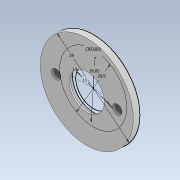
# Autodesk Inventor part: Sensor_AbstandFlansch
Saved by Autodesk Inventor 2022 (Build 260153000, 153)
## iProperties
Created: 2022-10-10
Part Number: Sensor_AbstandFlansch
Material: Generisch
Document SubType Name: Modeling
Designer: alexw
Density: 1 g/cm^3
Appearance: Vorgabe
Author: alexw
Autodesk Inventor part; units mm, degrees
ref_plane "YZ Plane" through (0, 0, 0) normal (1, 0, 0) x (0, 1, 0)
ref_plane "XZ Plane" through (0, 0, 0) normal (0, 1, 0) x (-1, 0, 0)
ref_plane "XY Plane" through (0, 0, 0) normal (0, 0, 1) x (1, 0, 0)
sketch "Skizze1" plane through (0, 0, 0) normal (0, 0, 1) x (1, 0, 0)
  circle A0 centre (0, 0) radius 14.5
  circle A1 centre (0, 0) radius 9.525 construction
  circle A2 centre (0, 0) radius 5.5
  circle A3 centre (0, 0) radius 6.5
  line L0 (-9.525, 0) -> (9.525, 0) construction
  circle A4 centre (0, 0) radius 10.45 construction
  line L1 (0, 0) -> (0, 10.45) construction
  point P0 (-9.05, -5.225)
  point P1 (9.05, -5.225)
  dimension "d15" = 20.9
  dimension "d0" = 29
  dimension "d1" = 19.05
  dimension "d2" = 11
  dimension "d3" = 13
  dimension "d18" = 360
  constraints: 5 coincident, 4 centre point, 4 end point, 2 point on circle, 1 horizontal, 1 midpoint, 1 vertical, 1 vertical alignment, 6 other
  measures "d0" diameter of A0
  measures "d1" diameter of A1
  measures "d2" diameter of A2
  measures "d3" diameter of A3
extrude "Extrusion1" add sketch "Skizze1" along normal blind 2 contours A0 | A3
extrude "Extrusion2" cut sketch "Skizze1" along normal blind 1.5 contours A3
hole "Bohrung1" at (-9.525, 0, 0) at (9.525, 0, 0) direction (0, 0, 1) diameter 2.9 end through all clearance for "Inbusschraube DIN EN ISO 4762" size "M2.5" standard "DIN"
